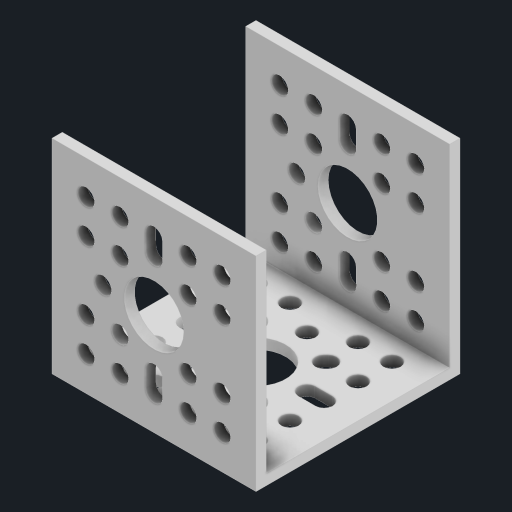
# Autodesk Inventor part: ShoulderServoBracket
Saved by Autodesk Inventor 2023 (Build 270158000, 158)
## iProperties
Created: 2021-01-26
Part Number: ShoulderServoBracket
Material: Generic
Document SubType Name: Modeling
Designer: valer
Density: 1 g/cm^3
Appearance: Default
Author: valer
Autodesk Inventor part; units mm, degrees
ref_plane "YZ Plane" through (0, 0, 0) normal (1, 0, 0) x (0, 1, 0)
ref_plane "XZ Plane" through (0, 0, 0) normal (0, 1, 0) x (-1, 0, 0)
ref_plane "XY Plane" through (0, 0, 0) normal (0, 0, 1) x (1, 0, 0)
sketch "Base" plane through (0, 0, 0) normal (0, 0, 1) x (1, 0, 0)
  line L0 (-24, 24) -> (24, 24)
  line L1 (24, 24) -> (24, -24)
  line L2 (24, -24) -> (-24, -24)
  line L3 (-24, -24) -> (-24, 24)
  line L4 (0, 24) -> (0, -24) construction
  line L5 (-24, 0) -> (24, 0) construction
  circle A0 centre (0, 0) radius 7
  circle A1 centre (0, 0) radius 12 construction
  line L6 (0, 12) -> (-12, 0) construction
  line L7 (-12, 0) -> (0, -12) construction
  line L8 (0, -12) -> (12, 0) construction
  line L9 (12, 0) -> (0, 12) construction
  line L10 (-24, 16) -> (24, 16) construction
  line L11 (-24, 8) -> (24, 8) construction
  line L12 (-24, -16) -> (24, -16) construction
  line L13 (-24, -8) -> (24, -8) construction
  line L14 (-16, 24) -> (-16, -24) construction
  line L15 (-8, 24) -> (-8, -24) construction
  line L16 (16, 24) -> (16, -24) construction
  line L17 (8, 24) -> (8, -24) construction
  circle A2 centre (-16, 16) radius 2
  circle A3 centre (-8, 16) radius 2
  circle A4 centre (-16, 8) radius 2
  circle A5 centre (-8, 8) radius 2
  circle A6 centre (-12, 0) radius 2
  circle A7 centre (0, 16) radius 2
  circle A8 centre (0, 12) radius 2
  line L18 (-2, 16) -> (-1.993043, 11.833333)
  line L19 (2, 16) -> (1.993043, 11.833333)
  line L20 (24, 8) -> (-24, 8) construction
  circle A9 centre (16, 16) radius 2
  circle A10 centre (8, 16) radius 2
  circle A11 centre (8, 8) radius 2
  circle A12 centre (16, 8) radius 2
  circle A13 centre (-16, -16) radius 2
  circle A14 centre (-8, -16) radius 2
  circle A15 centre (-16, -8) radius 2
  circle A16 centre (-8, -8) radius 2
  circle A17 centre (16, -16) radius 2
  circle A18 centre (8, -16) radius 2
  circle A19 centre (8, -8) radius 2
  circle A20 centre (16, -8) radius 2
  circle A21 centre (0, -16) radius 2
  circle A22 centre (0, -12) radius 2
  line L21 (-2, -16) -> (-1.993043, -11.833333)
  line L22 (2, -16) -> (1.993043, -11.833333)
  circle A23 centre (12, 0) radius 2
  point P0 (0, 0)
  point P1 (-1.993589, -12.160011)
  point P2 (1.993589, -12.160011)
  point P3 (1.993589, 12.160011)
  point P4 (-1.993589, 12.160011)
  dimension "d0" = 14
  dimension "d1" = 24
  dimension "d2" = 48
  dimension "d3" = 8
  dimension "d4" = 8
  dimension "d5" = 8
  dimension "d6" = 8
  dimension "d7" = 4
  constraints: 46 end point, 28 symmetric about line, 24 centre point, 21 point on line, 12 point on circle, 8 perpendicular, 7 equal radius, 6 coincident, 6 midpoint, 4 parallel, 1 horizontal, 14 other
  measures "d0" diameter of A0
  measures "d1" diameter of A1
  measures "d2" distance of L0.start L0.end
  measures "d3" distance between parallel lines of L0 L10
  measures "d4" distance between parallel lines of L11 L10
  measures "d5" distance between parallel lines of L3 L14
  measures "d6" distance between parallel lines of L14 L15
  measures "d7" diameter of A2
extrude "BaseFeature" add sketch "Base" along normal blind 2.43 contours L0 L1 L2 L3 | A23
sketch "Side" plane through (-24, -24, 0) normal (0, -1, 0) x (1, 0, 0)
  line L0 (0, 2.43) -> (48, 2.43) projected
  line L1 (48, 2.43) -> (0, 2.43)
  line L2 (0, 2.43) -> (0, -45.57)
  line L3 (0, -45.57) -> (48, -45.57)
  line L4 (48, -45.57) -> (48, 2.43)
  point P0 (24, 0)
  dimension "d10" = 48
  constraints: 8 end point, 2 parallel, 1 horizontal, 1 perpendicular
  measures "d10" distance of L3.end L0.end
extrude "SideFeature" add sketch "Side" against normal blind 2.43
sketch "Side2" plane through (-24, -24, 2.43) normal (0, -1, 0) x (1, 0, 0)
  line L0 (48, -48) -> (48, 0) construction
  line L1 (0, 0) -> (48, 0) construction
  line L2 (0, 0) -> (0, -48) construction
  line L3 (0, -48) -> (48, -48) construction
  line L4 (48, -48) -> (48, 0) construction
  line L5 (48, -24) -> (0, -24) construction
  line L6 (0, -48) -> (0, -2.43) construction
  line L7 (22, 0) -> (26, 0) construction
  line L8 (24, 0) -> (24, -48) construction
  circle A0 centre (24, -24) radius 7
  circle A1 centre (24, -24) radius 12 construction
  line L9 (48, -8) -> (0, -8) construction
  line L10 (48, -16) -> (0, -16) construction
  line L11 (48, -40) -> (0, -40) construction
  line L12 (48, -32) -> (0, -32) construction
  line L13 (40, 0) -> (40, -48) construction
  line L14 (0, 0) -> (48, 0)
  line L15 (32, 0) -> (32, -48) construction
  line L16 (8, 0) -> (8, -48) construction
  line L17 (16, 0) -> (16, -48) construction
  line L18 (36, -24) -> (24, -12) construction
  line L19 (12, -24) -> (24, -12) construction
  line L20 (36, -24) -> (24, -36) construction
  line L21 (12, -24) -> (24, -36) construction
  circle A2 centre (40, -8) radius 2
  circle A3 centre (40, -24) radius 2
  circle A4 centre (36, -24) radius 2
  circle A5 centre (40, -16) radius 2
  circle A6 centre (32, -8) radius 2
  circle A7 centre (24, -12) radius 2
  circle A8 centre (32, -16) radius 2
  circle A9 centre (32.485281, -15.514719) radius 2
  line L22 (32.485281, -15.514719) -> (24, -24) construction
  line L23 (33.899495, -16.928932) -> (33.414214, -17.414214)
  line L24 (31.071068, -14.100505) -> (30.585786, -14.585786)
  circle A10 centre (40, -40) radius 2
  circle A11 centre (40, -32) radius 2
  circle A12 centre (32, -40) radius 2
  circle A13 centre (32, -32) radius 2
  circle A14 centre (32.485281, -32.485281) radius 2
  line L25 (32.485281, -32.485281) -> (24, -24) construction
  line L26 (33.899495, -31.071068) -> (33.414214, -30.585786)
  line L27 (31.071068, -33.899495) -> (30.585786, -33.414214)
  circle A15 centre (24, -36) radius 2
  circle A16 centre (8, -8) radius 2
  circle A17 centre (8, -24) radius 2
  circle A18 centre (12, -24) radius 2
  circle A19 centre (8, -16) radius 2
  circle A20 centre (16, -8) radius 2
  circle A21 centre (16, -16) radius 2
  circle A22 centre (15.514719, -15.514719) radius 2
  circle A23 centre (8, -32) radius 2
  circle A24 centre (16, -40) radius 2
  circle A25 centre (8, -40) radius 2
  circle A26 centre (16, -32) radius 2
  circle A27 centre (15.514719, -32.485281) radius 2
  line L28 (40, -22) -> (35.833333, -22.006957)
  line L29 (40, -26) -> (35.833333, -25.993043)
  line L30 (12.166667, -22.006957) -> (8, -22)
  line L31 (12, -26) -> (8, -26)
  line L32 (16.928932, -14.100505) -> (17.414214, -14.585786)
  line L33 (14.585786, -17.414214) -> (14.100505, -16.928932)
  line L34 (17.414214, -33.414214) -> (16.928932, -33.899495)
  line L35 (14.585786, -30.585786) -> (14.100505, -31.071068)
  dimension "d19" = 24
  dimension "d18" = 14
  dimension "d20" = 8
  dimension "d21" = 8
  dimension "d22" = 8
  dimension "d23" = 8
  dimension "d24" = 4
  constraints: 56 end point, 29 point on line, 27 centre point, 24 point on circle, 23 symmetric about line, 16 tangent, 10 equal radius, 5 coincident, 5 midpoint, 5 perpendicular, 1 horizontal, 1 parallel, 26 other
  measures "d18" diameter of A0
  measures "d20" distance between parallel lines of L1 L9
  measures "d21" distance between parallel lines of L10 L9
  measures "d22" distance between parallel lines of L4 L13
  measures "d23" distance between parallel lines of L15 L13
  measures "d24" diameter of A2
sketch "Side2 outline for Side2Feature" plane through (-24, -24, 2.43) normal (0, -1, 0) x (1, 0, 0)
  line L0 (17.414214, -14.585786) -> (16.928932, -14.100505)
  arc A0 (14.585786, -17.414214) -> (17.414214, -14.585786) centre (16, -16) ccw
  line L1 (14.100505, -16.928932) -> (14.585786, -17.414214)
  arc A1 (16.928932, -14.100505) -> (14.100505, -16.928932) centre (15.514719, -15.514719) ccw
  line L2 (16.928932, -33.899495) -> (17.414214, -33.414214)
  arc A2 (14.100505, -31.071068) -> (16.928932, -33.899495) centre (15.514719, -32.485281) ccw
  line L3 (14.585786, -30.585786) -> (14.100505, -31.071068)
  arc A3 (17.414214, -33.414214) -> (14.585786, -30.585786) centre (16, -32) ccw
  circle A4 centre (16, -40) radius 2
  circle A5 centre (8, -40) radius 2
  circle A6 centre (8, -32) radius 2
  line L4 (12.166667, -22.006957) -> (8, -22)
  arc A7 (12, -26) -> (12.166667, -22.006957) centre (12, -24) ccw
  line L5 (8, -26) -> (12, -26)
  arc A8 (8, -22) -> (8, -26) centre (8, -24) ccw
  circle A9 centre (8, -16) radius 2
  circle A10 centre (8, -8) radius 2
  circle A11 centre (16, -8) radius 2
  circle A12 centre (24, -12) radius 2
  circle A13 centre (24, -36) radius 2
  circle A14 centre (32, -40) radius 2
  line L6 (30.585786, -33.414214) -> (31.071068, -33.899495)
  arc A15 (33.414214, -30.585786) -> (30.585786, -33.414214) centre (32, -32) ccw
  line L7 (33.899495, -31.071068) -> (33.414214, -30.585786)
  arc A16 (31.071068, -33.899495) -> (33.899495, -31.071068) centre (32.485281, -32.485281) ccw
  line L8 (31.071068, -14.100505) -> (30.585786, -14.585786)
  arc A17 (33.899495, -16.928932) -> (31.071068, -14.100505) centre (32.485281, -15.514719) ccw
  line L9 (33.414214, -17.414214) -> (33.899495, -16.928932)
  arc A18 (30.585786, -14.585786) -> (33.414214, -17.414214) centre (32, -16) ccw
  circle A19 centre (32, -8) radius 2
  circle A20 centre (40, -8) radius 2
  circle A21 centre (40, -16) radius 2
  arc A22 (40, -26) -> (40, -22) centre (40, -24) ccw
  line L10 (35.833333, -25.993043) -> (40, -26)
  arc A23 (35.833333, -22.006957) -> (35.833333, -25.993043) centre (36, -24) ccw
  line L11 (40, -22) -> (35.833333, -22.006957)
  circle A24 centre (40, -32) radius 2
  circle A25 centre (40, -40) radius 2
  circle A26 centre (24, -24) radius 7
extrude "Side2Feature" cut sketch "Side2 outline for Side2Feature" against normal blind 2.5
sketch "Sketch4" plane through (24, -24, -45.57) normal (0, 0, -1) x (-1, 0, 0)
  line L0 (0, 2.43) -> (48, 2.43)
  line L1 (48, 48) -> (48, 2.43)
  line L2 (0, 48) -> (48, 48)
  line L3 (0, 2.43) -> (0, 48)
  arc A0 (22, 8) -> (26, 8) centre (24, 8) ccw
  line L4 (22.006411, 11.839989) -> (22, 8)
  arc A1 (25.993589, 11.839989) -> (22.006411, 11.839989) centre (24, 12) ccw
  line L5 (26, 8) -> (25.993589, 11.839989)
  circle A2 centre (8, 16) radius 2
  circle A3 centre (16, 8) radius 2
  circle A4 centre (40, 16) radius 2
  circle A5 centre (8, 32) radius 2
  circle A6 centre (16, 40) radius 2
  circle A7 centre (8, 40) radius 2
  arc A8 (22.006411, 36.160011) -> (25.993589, 36.160011) centre (24, 36) ccw
  line L6 (22, 40) -> (22.006411, 36.160011)
  arc A9 (26, 40) -> (22, 40) centre (24, 40) ccw
  line L7 (25.993589, 36.160011) -> (26, 40)
  circle A10 centre (40, 40) radius 2
  circle A11 centre (32, 40) radius 2
  circle A12 centre (40, 32) radius 2
  circle A13 centre (36, 24) radius 2
  circle A14 centre (40, 8) radius 2
  circle A15 centre (32, 8) radius 2
  circle A16 centre (8, 8) radius 2
  circle A17 centre (32, 32) radius 2
  circle A18 centre (16, 32) radius 2
  circle A19 centre (16, 16) radius 2
  circle A20 centre (32, 16) radius 2
  circle A21 centre (24, 24) radius 7
extrude "Extrusion4" add sketch "Sketch4" against normal blind 2.43
body "Solid1"
